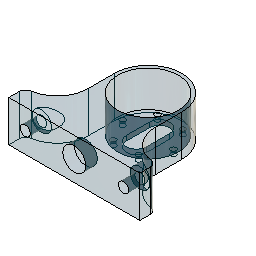
Support_Moteur (Autodesk Fusion 360 design; units mm, degrees)
Autodesk Fusion 360 part; units mm, degrees
sketch "Sketch1" plane through (0, 0, 0) normal (0, 0, 1) x (1, 0, 0)
  circle A0 centre (0, 0) radius 15.5 construction
  circle A1 centre (0, 0) radius 18.5
  circle A2 centre (0, 0) radius 20.5
  line L0 (-18.5, 0) -> (18.5, 0) construction
  circle A3 centre (-15.5, 0) radius 1.6
  circle A4 centre (15.5, 0) radius 1.6
  circle A5 centre (7.75, -13.4234) radius 1.6
  circle A6 centre (-7.75, -13.4234) radius 1.6
  circle A7 centre (7.75, 13.4234) radius 1.6
  circle A8 centre (-7.75, 13.4234) radius 1.6
  line L1 (0, 18.5) -> (0, -40) construction
  line L2 (40, -45) -> (-40, -45)
  line L3 (-40, -45) -> (-40, -35)
  line L4 (-40, -35) -> (40, -35)
  line L5 (40, -35) -> (40, -45)
  line L6 (40, -45) -> (-40, -35) construction
  line L7 (-40, -45) -> (40, -35) construction
  line L8 (-20.5, -35) -> (-20.5, 0)
  line L9 (20.5, -35) -> (20.5, 0)
  circle A9 centre (0, 7) radius 6.1
  circle A10 centre (0, -7) radius 6.1
  line L10 (-6.1, -7) -> (-6.1, 7)
  line L11 (6.1, 7) -> (6.1, -7)
  dimension "d1" = 31
  dimension "d2" = 37
  dimension "d3" = 2
  dimension "d4" = 3.2
  dimension "d5" = 3.2
  dimension "d6" = 3.2
  dimension "d7" = 3.2
  dimension "d8" = 3.2
  dimension "d9" = 3.2
  dimension "d10" = 15.5
  dimension "d11" = 15.5
  dimension "d12" = 15.5
  dimension "d13" = 15.5
  dimension "d14" = 15.5
  dimension "d21" = 10
  dimension "d22" = 80
  dimension "d32" = 12.2
  dimension "d33" = 7
  dimension "d52" = 35
  constraint coincident A0.centre A1.centre
  constraint concentric A0 A1
  constraint horizontal L0
  constraint coincident A1 L0.end
  constraint coincident A1 L0.start
  constraint coincident A0.centre L0
  constraint coincident A0 A3.centre
  constraint coincident L0 A3.centre
  constraint coincident A0 A4.centre
  constraint coincident L0 A4.centre
  constraint coincident A0 A5.centre
  constraint coincident A0 A6.centre
  constraint coincident A0 A7.centre
  constraint coincident A0 A8.centre
  constraint coincident A1 L1.start
  constraint perpendicular L0 L1
  constraint perpendicular L2 L3
  constraint parallel L2 L4
  constraint parallel L3 L5
  constraint horizontal L2
  constraint coincident A0.centre L1
  constraint midpoint L1.end L7
  constraint coincident L4 L8.start
  constraint coincident A2 L8.end
  constraint tangent A2 L8
  constraint perpendicular L4 L8
  constraint coincident L4 L9.start
  constraint coincident A2 L9.end
  constraint tangent A2 L9
  constraint perpendicular L4 L9
  constraint coincident L1 A9.centre
  constraint symmetric L0 A9 A10
  constraint coincident A10 L10.start
  constraint coincident A9 L10.end
  constraint tangent A9 L10
  constraint coincident A9 L11.start
  constraint coincident A10 L11.end
  constraint tangent A10 L11
  constraint tangent A9 L11
  constraint tangent A10 L10
  measures "d1" diameter of A0
  measures "d2" diameter of A1
  measures "d3" distance of A1 A2
  measures "d4" diameter of A3
  measures "d5" diameter of A4
  measures "d6" diameter of A5
  measures "d7" diameter of A6
  measures "d8" diameter of A7
  measures "d9" diameter of A8
  measures "d10" distance of A3.centre A6.centre
  measures "d11" distance of A4.centre A5.centre
  measures "d12" distance of A5.centre A6.centre
  measures "d13" distance of A4.centre A7.centre
  measures "d14" distance of A3.centre A8.centre
  measures "d21" distance of L2.end L3.end
  measures "d22" distance of L2.start L2.end
  measures "d32" diameter of A9
  measures "d33" distance of A0.centre A9.centre
  measures "d52" vertical distance of A0.centre L4.end
extrude "Extrude1" add sketch "Sketch1" along normal blind 3 contours A1
extrude "Extrude2" add sketch "Sketch1" along normal blind 25 contours A2 | A2 L4 L8 L9 | L2 L3 L4 L5
sketch "Sketch6" plane through (0, -35, 0) normal (0, 1, 0) x (-1, 0, 0)
  line L0 (20.5, 0) -> (40, 0)
  line L1 (40, 0) -> (40, 25)
  line L2 (40, 25) -> (20.5, 25)
  line L3 (20.5, 25) -> (20.5, 0)
  line L4 (-40, 0) -> (-20.5, 0)
  line L5 (-20.5, 0) -> (-20.5, 25)
  line L6 (-20.5, 25) -> (-40, 25)
  line L7 (-40, 25) -> (-40, 0)
  line L8 (-40, 12.5) -> (40, 12.5) construction
  circle A0 centre (-30, 12.5) radius 3.1
  line L9 (0, 0) -> (0, 42.7428) construction
  circle A1 centre (30, 12.5) radius 3.1
  circle A2 centre (30, 12.5) radius 6
  circle A3 centre (-30, 12.5) radius 6
  dimension "d42" = 6.2
  dimension "d43" = 6.2
  dimension "d44" = 30
  dimension "d45" = 30
  dimension "d46" = 12
  dimension "d47" = 12
  constraint midpoint L7 L8.start
  constraint midpoint L1 L8.end
  constraint coincident L8 A0.centre
  constraint coincident L9.start origin
  constraint perpendicular L8 L9
  constraint coincident L8 A1.centre
  constraint concentric A1 A2
  constraint concentric A0 A3
  measures "d42" diameter of A0
  measures "d43" diameter of A1
  measures "d44" horizontal distance of L9.start A0.centre
  measures "d45" horizontal distance of L9.start A1.centre
  measures "d46" diameter of A2
  measures "d47" diameter of A3
fillet "Fillet2" radius 19 2 edges at (20.5, -35, 12.5) (-20.5, -35, 12.5)
extrude "Extrude3" cut sketch "Sketch6" against normal through all contours A0 | A1
extrude "Extrude4" cut sketch "Sketch6" along normal through all contours A0 | A1 | A2 | A3
fillet "Fillet3" radius 4 2 edges at (40, -35, 12.5) (-40, -35, 12.5)
sketch "Sketch7" plane through (0, -45, 0) normal (0, -1, 0) x (1, 0, 0)
  circle A0 centre (30, 12.5) radius 3.1
  circle A1 centre (-30, 12.5) radius 3.1
  line L0 (-40, 0) -> (40, 0)
  line L1 (40, 0) -> (40, 25)
  line L2 (40, 25) -> (-40, 25)
  line L3 (-40, 25) -> (-40, 0)
  line L4 (-30, 12.5) -> (30, 12.5) construction
  circle A2 centre (0, 12.5) radius 7
  dimension "d55" = 14
  constraint coincident A1.centre L4.start
  constraint coincident A0.centre L4.end
  constraint midpoint L4 A2.centre
  measures "d55" diameter of A2
extrude "Extrude7" cut sketch "Sketch7" against normal blind 7 contours A2
named bodies: "Support_D37"
